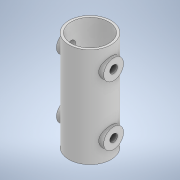
# Autodesk Inventor part: Lot_Truot
Saved by Autodesk Inventor 2022 (Build 260153000, 153)
## iProperties
Created: 2022-11-18
Part Number: Lot_Truot
Material: Generic
Document SubType Name: Modeling
Designer: nguye
Density: 1 g/cm^3
Appearance: Default
Author: nguye
Autodesk Inventor part; units mm, degrees
ref_plane "XZ Plane" through (0, 0, 0) normal (0, 1, 0) x (-1, 0, 0)
ref_plane "XY Plane" through (0, 0, 0) normal (0, 0, 1) x (1, 0, 0)
sketch "Sketch1" plane through (0, 0, 0) normal (0, 1, 0) x (-1, 0, 0)
  circle A0 centre (0, 0) radius 7.55
  circle A1 centre (0, 0) radius 8.5
  dimension "d0" = 15.1
  dimension "d1" = 17
  constraints: 2 centre point, 2 coincident
  measures "d0" diameter of A0
  measures "d1" diameter of A1
extrude "Extrusion1" add sketch "Sketch1" along normal blind 40
ref_plane "Work Plane1" through (9, 0, 0) normal (1, 0, 0) x (0, 1, 0)
sketch "Sketch2" plane through (9, 0, 0) normal (1, 0, 0) x (0, 1, 0)
  circle A0 centre (32, 0) radius 4
  circle A1 centre (8, 0) radius 4
  point P0 (0, 0)
  dimension "d5" = 8
  dimension "d6" = 24
  dimension "d7" = 8
  constraints: 2 centre point, 2 horizontal alignment, 1 equal radius
  measures "d5" distance of point (0, 0) A1.centre
  measures "d6" distance of A0.centre A1.centre
  measures "d7" diameter of A0
extrude "Extrusion2" add sketch "Sketch2" along normal up to surface round surface about axis through (0, 0, 0) along (0, 1, 0) radius 8.5 far side no
extrude "Extrusion3" add sketch "Sketch2" along normal blind 0.5 from surface at 0
sketch "Sketch3" plane through (9.5, 32, 0) normal (1, 0, 0) x (0, 0, -1)
  circle A0 centre (0, 0) radius 4 projected
  circle A1 centre (0, -24) radius 4 projected
  point P0 (0, -32)
  constraints: 2 coincident
hole "Hole1" at (9.5, 32, 0) at (9.5, 8, 0) direction (-1, 0, 0) diameter 3.1 end up to surface
mirror "Mirror1" about plane through (0, 0, 0) normal (1, 0, 0) of "Extrusion3", "Hole1", "Extrusion2"
body "Solid1"
